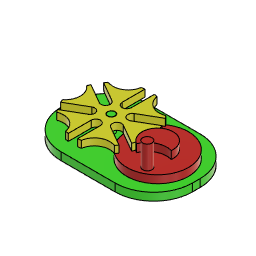
6 slots geneva (Autodesk Fusion 360 design; units mm, degrees)
Autodesk Fusion 360 part; units mm, degrees
sketch "Holder" plane through (0, 0, 0) normal (0, 0, 1) x (1, 0, 0) in component "Holder"
  line L0 (85, 55) -> (-85, 55)
  line L1 (-85, 55) -> (-85, -55)
  line L2 (-85, -55) -> (85, -55)
  line L3 (85, -55) -> (85, 55)
  line L4 (85, 55) -> (-85, -55) construction
  line L5 (-85, 55) -> (85, -55) construction
  line L6 (-85, -55) -> (-25, -55) construction
  line L7 (-25, -55) -> (85, -55) construction
  line L8 (-85, 0) -> (85, 0) construction
  dimension "d1" = 170
  dimension "d2" = 110
  dimension "d3" = 60
  constraint horizontal L0
  constraint perpendicular L0 L1
  constraint parallel L0 L2
  constraint parallel L1 L3
  constraint coincident L4 origin
  constraint coincident L5 origin
  constraint perpendicular L1 L6
  constraint midpoint L1 L8.start
  constraint midpoint L3 L8.end
  measures "d1" distance of L1.end L2.end
  measures "d2" distance of L0.end L1.end
  measures "d3" distance of L1.end L6.end
extrude "Extrude1" add sketch "Holder" along normal blind 10 makes body 1 in component "Holder"
sketch "Circle with pin" plane through (0, 0, 10) normal (0, 0, 1) x (-1, 0, 0) in component "Circle with pin"
  line L0 (-85, 55) -> (-85, -55)
  line L1 (-85, -55) -> (85, -55)
  line L2 (85, -55) -> (85, 55)
  line L3 (85, 55) -> (-85, 55)
  line L4 (85, 55) -> (-35, 55) construction
  line L5 (-35, 55) -> (-35, 0) construction
  circle A0 centre (-35, 0) radius 40
  circle A1 centre (-35, 0) radius 20
  circle A2 centre (-17.6167, -23.7048) radius 6
  circle A3 centre (-17.6167, -23.7048) radius 25
  circle A4 centre (-35, 0) radius 4
  dimension "d6" = 120
  dimension "d7" = 80
  dimension "d8" = 40
  dimension "d9" = 12
  dimension "d10" = 50
  dimension "d17" = 8
  constraint coincident L2.end L3.start
  constraint perpendicular L2 L4
  constraint perpendicular L4 L5
  constraint coincident L5.end A0.centre
  constraint concentric A0 A1
  constraint concentric A2 A3
  measures "d6" distance of L2.end L4.end
  measures "d7" diameter of A0
  measures "d8" diameter of A1
  measures "d9" diameter of A2
  measures "d10" diameter of A3
  measures "d17" diameter of A4
extrude "Extrude2" add sketch "Circle with pin" along normal blind 20 separate body contours A1 A3 | A4 picked at (-25.1554, 5.9598) makes body 2 in component "Circle with pin"
extrude "Extrude1'" add sketch "Circle with pin" along normal blind 10 separate body contours A0 A1 A3 | A0 A1 A3 | A1 A3 | A1 A3 | A4 makes body 3 in component "Circle with pin"
extrude "Extrude3" add sketch "Circle with pin" along normal blind 40 contours A2 bodies 3 in component "Circle with pin"
combine "Combine1" operation add target body 2 tool bodies 3 in component "Circle with pin"
extrude "Extrude4" cut sketch "Circle with pin" along normal blind 10 contours A4 bodies 2 in component "Circle with pin"
extrude "Extrude2'" add sketch "Circle with pin" along normal blind 10 contours A4 bodies 1 in component "Holder"
move_face "OffsetFaces1" offset -0.2 1 faces at (31.005, 0.1994, 16.6667) on bodies 1 in component "Holder"
sketch "Circle with slots" plane through (0, 0, 10) normal (0, 0, 1) x (-1, 0, 0) in component "Circle with slots"
  line L0 (85, 55, 11) -> (25, 55, 11) construction
  line L1 (25, 55, 11) -> (25, 0, 11) construction
  circle A0 through (75, 0, 11) (0, 43.3013, 11) (0, -43.3013, 11)
  line L2 (25, 0, 11) -> (25, -50, 11) construction
  line L3 (25, 0, 11) -> (19, 0, 11) construction
  line L4 (19, 0, 11) -> (19, -49.6387, 11) construction
  line L5 (25, 0, 11) -> (25, -20, 11) construction
  circle A1 through (31, -20, 11) (22, -14.8038, 11) (22, -25.1962, 11)
  line L6 (19, -49.6387, 11) -> (19, 0, 11)
  line L7 (31, -49.6387, 11) -> (31, 0, 11)
  line L8 (64.9884, -30.0155, 11) -> (22, -5.1962, 11)
  line L9 (70.9884, -19.6232, 11) -> (28, 5.1962, 11)
  circle A2 through (48.3205, -10, 11) (39.3205, -4.8038, 11) (39.3205, -15.1962, 11)
  line L10 (70.9884, 19.6232, 11) -> (28, -5.1962, 11)
  line L11 (64.9884, 30.0155, 11) -> (22, 5.1962, 11)
  circle A3 through (48.3205, 10, 11) (39.3205, 15.1962, 11) (39.3205, 4.8038, 11)
  line L12 (31, 49.6387, 11) -> (31, 0, 11)
  line L13 (19, 49.6387, 11) -> (19, 0, 11)
  circle A4 through (31, 20, 11) (22, 25.1962, 11) (22, 14.8038, 11)
  line L14 (-14.9884, 30.0155, 11) -> (28, 5.1962, 11)
  line L15 (-20.9884, 19.6232, 11) -> (22, -5.1962, 11)
  circle A5 through (13.6795, 10, 11) (4.6795, 15.1962, 11) (4.6795, 4.8038, 11)
  line L16 (-20.9884, -19.6232, 11) -> (22, 5.1962, 11)
  line L17 (-14.9884, -30.0155, 11) -> (28, -5.1962, 11)
  circle A6 through (13.6795, -10, 11) (4.6795, -4.8038, 11) (4.6795, -15.1962, 11)
  circle A7 through (-15, 0, 11) (-45, 17.3205, 11) (-45, -17.3205, 11)
  line L18 (-22.5, -15.6125, 11) -> (-22.5, 15.6125, 11) construction
  circle A8 through (15, -51.9615, 11) (-15, -34.641, 11) (-15, -69.282, 11)
  circle A9 through (75, -51.9615, 11) (45, -34.641, 11) (45, -69.282, 11)
  circle A10 through (105, 0, 11) (75, 17.3205, 11) (75, -17.3205, 11)
  circle A11 through (75, 51.9615, 11) (45, 69.282, 11) (45, 34.641, 11)
  circle A12 through (15, 51.9615, 11) (-15, 69.282, 11) (-15, 34.641, 11)
  circle A13 through (30, 0, 11) (22.5, 4.3301, 11) (22.5, -4.3301, 11)
  dimension "d27" = 60
  dimension "d28" = 100
  dimension "d29" = 6
  dimension "d30" = 12
  dimension "d35" = 10
extrude "Extrude1''" add sketch "Circle with slots" along normal blind 9 separate body contours A0 L9 L10 A10 | A0 L11 L12 A11 | L9 L10 L11 A3 L12 | L7 L9 L10 L12 | L7 L8 L9 A2 L10 | L9 L11 L12 L14 | L11 L12 L13 A4 L14 | L6 L7 L8 L9 L10 L11 L12 L13 L14 L15 L16 L17 | L7 L8 L10 L17 | L11 L13 L14 L16 | A0 L7 L8 A9 | A1 L6 L7 L8 L17 | A0 L13 L14 A12 | L13 L14 L15 A5 L16 | L6 L8 L15 L17 | L6 L13 L15 L16 | A0 L6 L17 A8 | L6 L15 L16 L17 A6 | A0 L15 L16 A7 | A13 in plane through (0, 0, 21) normal (0, 0, 1) makes body 4 in component "Circle with slots"
extrude "Extrude2''" cut sketch "Circle with slots" along normal blind 9 contours A13 in plane through (0, 0, 21) normal (0, 0, 1) bodies 4 in component "Circle with slots"
extrude "Extrude3'" add sketch "Circle with slots" along normal blind 9 and the other way blind 11 contours A13 in plane through (0, 0, 21) normal (0, 0, 1) bodies 1 in component "Holder"
move_face "OffsetFaces2" offset -0.3 1 faces at (-29.9938, 0.2492, 16.6667) on bodies 1 in component "Holder"
fillet "Fillet1" radius 50 4 edges at (85, -55, 5) (-85, -55, 5) (-85, 55, 5) (85, 55, 5) on bodies 1 in component "Holder"
component "Holder" placed x (1, 0, 0) y (0, 1, 0) z (0, 0, 1) at (0, 0, 0)
component "Circle with pin" placed x (1, 0, 0) y (0, 1, 0) z (0, 0, 1) at (0, 0, 0)
component "Circle with slots" placed x (1, 0, 0) y (0, 1, 0) z (0, 0, 1) at (0, 0, 0)
named bodies: "Holder", "Circle with pin", "Circle with slots"
